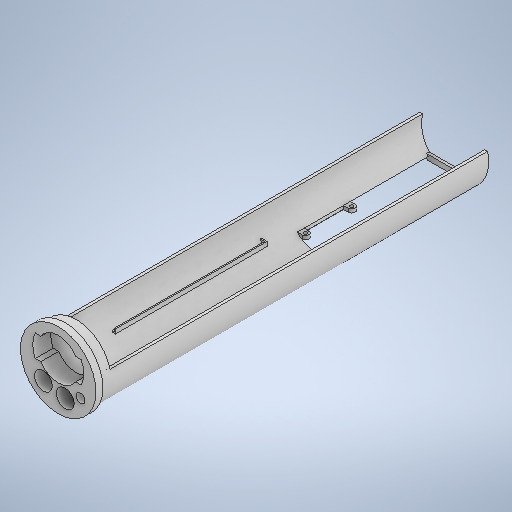
# Autodesk Inventor part: PCB tray CAD
Saved by Autodesk Inventor 2025 (Build 290162000, 162)
## iProperties
Created: 2024-07-01
Part Number: PCB tray CAD
Material: Generic
Document SubType Name: Modeling
Designer: track
Density: 1 g/cm^3
Appearance: Default
Author: track
## iProperties of the stored document PCB tray CAD_3DPrint.ipt
Created: 2024-07-01
Part Number: PCB tray CAD_3DPrint
Material: Generic
Document SubType Name: Modeling
Designer: track
Density: 1 g/cm^3
Appearance: Default
Author: track
Autodesk Inventor part; units mm, degrees
ref_plane "YZ Plane" through (0, 0, 0) normal (1, 0, 0) x (0, 1, 0)
ref_plane "XY Plane" through (0, 0, 0) normal (0, 0, 1) x (1, 0, 0)
sketch "Sketch9" plane through (0, 0, 0) normal (0, 0, 1) x (1, 0, 0)
  circle A0 centre (0, 0) radius 25.4
  circle A1 centre (0, 0) radius 23.4
  dimension "d29" = 50.8
  dimension "d30" = 2
  constraints: 2 centre point, 2 coincident
  measures "d29" diameter of A0
  measures "d30" radial gap between concentric circles of A0 A1
extrude "Extrusion7" add sketch "Sketch9" against normal blind 287
sketch "Sketch10" plane through (0, 0, 0) normal (0, 0, 1) x (1, 0, 0)
  circle A0 centre (-10.795, -12.065) radius 6.5
  circle A1 centre (5.08, -15.24) radius 6.55
  circle A2 centre (16.129, -9.525) radius 3.3
  circle A3 centre (0, 0) radius 23.4 projected
  line L0 (17.25, -1.015) -> (-17.25, -1.015) construction
  line L1 (-17.25, -1.015) -> (-17.25, 14.985) construction
  line L2 (-17.25, 14.985) -> (17.25, 14.985) construction
  line L3 (17.25, 14.985) -> (17.25, -1.015) construction
  line L4 (17.25, -1.015) -> (-17.25, 14.985) construction
  line L5 (-17.25, -1.015) -> (17.25, 14.985) construction
  arc A4 (-12.6886, -1.015) -> (12.6886, -1.015) centre (0, 6.985) ccw
  arc A5 (12.6886, 14.985) -> (-12.6886, 14.985) centre (0, 6.985) ccw
  circle A6 centre (0, 6.985) radius 18.5 construction
  arc A7 (16.6808, -1.015) -> (16.6808, 14.985) centre (0, 6.985) ccw
  arc A8 (-16.6808, 14.985) -> (-16.6808, -1.015) centre (0, 6.985) ccw
  line L6 (-16.6808, 14.985) -> (-12.6886, 14.985)
  line L7 (12.6886, 14.985) -> (16.6808, 14.985)
  line L8 (16.6808, -1.015) -> (12.6886, -1.015)
  line L9 (-12.6886, -1.015) -> (-16.6808, -1.015)
  point P0 (18.5865, 14.2162)
  point P1 (17.7647, -15.2307)
  dimension "d33" = 13
  dimension "d34" = 13.1
  dimension "d35" = 6.6
  dimension "d90" = 16
  dimension "d91" = 34.5
  dimension "d92" = 15
  dimension "d93" = 15
  dimension "d94" = 37
  dimension "d95" = 0
  dimension "d96" = 6.985
  dimension "d97" = 9.525
  dimension "d98" = 16.129
  dimension "d99" = 5.08
  dimension "d100" = 15.24
  dimension "d101" = 10.795
  dimension "d102" = 12.065
  constraints: 20 end point, 12 point on circle, 8 centre point, 8 point on line, 3 collinear, 3 parallel, 2 concentric, 2 midpoint, 1 coincident, 1 horizontal, 1 perpendicular
  measures "d33" diameter of A0
  measures "d34" diameter of A1
  measures "d35" diameter of A2
  measures "d90" distance between parallel lines of L2 L0
  measures "d91" distance of L1.end L2.end
  measures "d92" radius of A5
  measures "d93" radius of A4
  measures "d94" diameter of A6
  measures "d95" horizontal distance of point (0, 0) A4.centre
  measures "d96" distance of A4.centre point (0, 0)
  measures "d97" vertical distance of A2.centre point (0, 0)
  measures "d98" horizontal distance of point (0, 0) A2.centre
  measures "d99" horizontal distance of point (0, 0) A1.centre
  measures "d100" vertical distance of A3.centre A1.centre
  measures "d101" horizontal distance of point (0, 0) A0.centre
  measures "d102" vertical distance of point (0, 0) A0.centre
extrude "Extrusion8" add sketch "Sketch10" against normal blind 13
ref_plane "Work Plane1" through (0, 25.4, 0) normal (0, 1, 0) x (-1, 0, 0)
sketch "Sketch11" plane through (0, 25.4, 0) normal (0, 1, 0) x (-1, 0, 0)
  line L0 (-25.4, -287) -> (25.4, -287) projected
  line L1 (-25.4, 0) -> (-25.4, -287) projected
  line L2 (25.4, -287) -> (-25.4, -287)
  line L3 (-25.4, -287) -> (-25.4, -190)
  line L4 (-25.4, -190) -> (25.4, -190)
  line L5 (25.4, -190) -> (25.4, -287)
  point P0 (0, 0)
  dimension "d53" = 97
  constraints: 8 end point, 2 parallel, 1 horizontal, 1 perpendicular, 1 point on line
  measures "d53" distance of L4.end L0.end
extrude "Extrusion9" cut sketch "Sketch11" against normal blind 19.05
sketch "Sketch12" plane through (0, 0, -287) normal (0, 0, -1) x (-1, 0, 0)
  circle A0 centre (0, 0) radius 25.4 projected
  line L0 (-19.2809, -16.535) -> (19.2809, -16.535)
  line L1 (16, -16.535) -> (-16, -16.535) projected
  arc A1 (-19.2809, -16.535) -> (19.2809, -16.535) centre (0, 0) ccw
  dimension "d86" = 16.535
  constraints: 4 point on circle, 2 end point, 1 centre point, 1 concentric, 1 horizontal
  measures "d86" distance from line of A0.centre L0
extrude "Extrusion10" cut sketch "Sketch12" against normal blind 97 contours L0 A0 picked at (1.0399, -19.4259)
ref_plane "Work Plane3" through (0, -16.51, 0) normal (0, 1, 0) x (-1, 0, 0)
sketch "Sketch13" plane through (0, -16.51, 0) normal (0, 1, 0) x (-1, 0, 0)
  line L0 (0, 0) -> (0, -257.1233) construction
  line L1 (-16.5576, -287) -> (-16.5576, -190) projected
  line L2 (-16.5576, -190) -> (-13.0576, -190)
  line L3 (-13.0576, -190) -> (-13.0576, -195) construction
  line L4 (-13.0576, -195) -> (-16.5576, -195)
  line L5 (-16.5576, -195) -> (-16.5576, -190)
  line L6 (16.5576, -190) -> (16.5576, -287) projected
  line L7 (16.5576, -190) -> (13.0576, -190)
  line L8 (13.0576, -190) -> (13.0576, -195) construction
  line L9 (13.0576, -195) -> (16.5576, -195)
  line L10 (16.5576, -195) -> (16.5576, -190)
  line L11 (-16.5576, -223.5) -> (-13.0576, -223.5)
  line L12 (-13.0576, -223.5) -> (-13.0576, -228.5) construction
  line L13 (-13.0576, -228.5) -> (-16.5576, -228.5)
  line L14 (-16.5576, -228.5) -> (-16.5576, -223.5)
  line L15 (16.5576, -223.5) -> (13.0576, -223.5)
  line L16 (13.0576, -223.5) -> (13.0576, -228.5) construction
  line L17 (13.0576, -228.5) -> (16.5576, -228.5)
  line L18 (16.5576, -228.5) -> (16.5576, -223.5)
  arc A0 (-13.0576, -195) -> (-13.0576, -190) centre (-13.0576, -192.5) ccw
  arc A1 (13.0576, -190) -> (13.0576, -195) centre (13.0576, -192.5) ccw
  arc A2 (-13.0576, -228.5) -> (-13.0576, -223.5) centre (-13.0576, -226) ccw
  arc A3 (13.0576, -223.5) -> (13.0576, -228.5) centre (13.0576, -226) ccw
  circle A4 centre (-13.0576, -192.5) radius 1.25
  circle A5 centre (13.0576, -192.5) radius 1.25
  circle A6 centre (-13.0576, -226) radius 1.25
  circle A7 centre (13.0576, -226) radius 1.25
  point P0 (-10.5576, -192.5)
  point P1 (16.5576, -228.5)
  point P2 (16.5576, -223.5)
  point P3 (-16.5576, -223.5)
  point P4 (-16.5576, -228.5)
  dimension "d60" = 5
  dimension "d61" = 5
  dimension "d62" = 28.5
  dimension "d63" = 6
  dimension "d64" = 2.5
  dimension "d65" = 2.5
  constraints: 34 end point, 9 point on circle, 8 centre point, 8 parallel, 8 tangent, 5 point on line, 4 coincident, 4 horizontal, 4 perpendicular, 1 vertical, 6 other
  measures "d60" distance of L2.end L3.end
  measures "d61" distance of L11.end L12.end
  measures "d62" distance between parallel lines of L4 L11
  measures "d63" distance from line of L1 point (-10.558, -192.5)
  measures "d64" diameter of A4
  measures "d65" diameter of A6
extrude "Extrusion11" add sketch "Sketch13" against normal blind 2.54
sketch "Sketch14" plane through (0, 0, -190) normal (0, 0, -1) x (-1, 0, 0)
  line L0 (16.5576, -19.05) -> (13.5889, -19.05) projected
  arc A0 (-13.5889, -19.05) -> (13.5889, -19.05) centre (0, 0) ccw projected
  line L1 (-13.5889, -19.05) -> (-16.5576, -19.05) projected
  line L2 (-16.5576, -19.05) -> (-16.5576, -16.535) projected
  line L3 (-19.2809, -16.535) -> (-16.5576, -16.535) projected
  arc A1 (-19.2809, -16.535) -> (19.2809, -16.535) centre (0, 0) ccw projected
  line L4 (16.5576, -16.535) -> (19.2809, -16.535) projected
  line L5 (16.5576, -16.535) -> (16.5576, -19.05) projected
  line L6 (13.0576, -16.51) -> (13.0576, -19.05) projected
  line L7 (13.0576, -19.05) -> (16.8005, -19.05)
  line L8 (-13.0576, -16.51) -> (-13.0576, -19.05) projected
  line L9 (-13.0576, -19.05) -> (-16.8005, -19.05)
  point P0 (-16.5576, -19.2615)
  point P1 (16.5576, -19.2615)
  constraints: 4 end point, 4 point on circle, 3 point on line, 1 perpendicular
extrude "Extrusion12" add sketch "Sketch14" along normal up to surface (38.5 mm away) contours L5 L4 A1 L7 | A1 L3 L2 L9
sketch "Sketch15" plane through (0, 25.4, 0) normal (0, 1, 0) x (-1, 0, 0)
  line L0 (-25.4, 0) -> (-25.4, -287) projected
  line L1 (25.4, 0) -> (25.4, -287) projected
  line L2 (-25.4, -13) -> (25.4, -13)
  line L3 (25.4, -13) -> (25.4, -193)
  line L4 (25.4, -193) -> (-25.4, -193)
  line L5 (-25.4, -193) -> (-25.4, -13)
  line L6 (23.4, -13) -> (-23.4, -13) projected
  point P0 (0, 0)
  point P1 (-25.4, -193)
  point P2 (25.4, -13)
  dimension "d70" = 0
  dimension "d71" = 180
  constraints: 8 end point, 2 parallel, 2 point on line, 1 horizontal, 1 perpendicular
  measures "d70" distance between parallel lines of L6 L2
  measures "d71" distance between parallel lines of L2 L4
extrude "Extrusion13" cut sketch "Sketch15" against normal up to surface (19.05 mm away)
sketch "Sketch17" plane through (0, 0, -287) normal (0, 0, -1) x (-1, 0, 0)
  circle A0 centre (0, 0) radius 25.4
  arc A1 (-16.8005, -19.05) -> (16.8005, -19.05) centre (0, 0) ccw projected
  line L0 (-19.2809, -16.535) -> (-16.5576, -16.535) projected
  line L1 (-20.32, -15.24) -> (20.32, -15.24)
  line L2 (16.5576, -19.05) -> (13.0576, -19.05) projected
  line L3 (-16.8005, -19.05) -> (16.8005, -19.05)
  point P0 (16.8005, -19.05)
  dimension "d74" = 3.81
  constraints: 4 end point, 2 parallel, 2 point on circle, 1 centre point, 1 coincident, 1 concentric
  measures "d74" distance between parallel lines of L1 L3
extrude "Extrusion14" add sketch "Sketch17" against normal blind 2 contours L1 A0 L3 L2
sketch "Sketch18" plane through (0, 0, -13) normal (0, 0, -1) x (-1, 0, 0)
  circle A0 centre (0, 0) radius 27.4
  circle A1 centre (0, 0) radius 25.4
  arc A2 (16.8005, -19.05) -> (24.5934, 6.35) centre (0, 0) ccw projected
  dimension "d87" = 2
  constraints: 2 centre point, 2 coincident, 1 concentric
  measures "d87" radial gap between concentric circles of A0 A1
extrude "Extrusion15" add sketch "Sketch18" along normal blind 5 from surface at -13
sketch "Sketch20" plane through (0, 0, -13) normal (0, 0, -1) x (-1, 0, 0)
  arc A0 (-22.5219, 6.35) -> (-17.7568, -15.24) centre (0, 0) ccw projected
  line L0 (-20.4714, -11.335) -> (20.4714, -11.335) construction
  arc A1 (-22.5219, 6.35) -> (22.5219, 6.35) centre (0, 0) ccw projected
  arc A2 (24.5934, 6.35) -> (-24.5934, 6.35) centre (0, 0) ccw projected
  line L1 (0, -23.4) -> (0, 25.4) construction
  line L2 (-16.4531, -11.335) -> (-17.3421, -11.335)
  line L3 (-17.3421, -11.335) -> (-17.3421, -13.621)
  line L4 (-17.3421, -13.621) -> (-19.027, -13.621)
  line L5 (-16.4531, -11.335) -> (-16.4531, -14.51)
  line L6 (-16.4531, -14.51) -> (-18.3581, -14.51)
  circle A3 centre (0, 0) radius 23.4
  line L7 (20.4714, -11.335) -> (-20.4714, -11.335) construction
  line L8 (16.4531, -11.335) -> (17.3421, -11.335)
  line L9 (17.3421, -11.335) -> (17.3421, -13.621)
  line L10 (17.3421, -13.621) -> (19.027, -13.621)
  line L11 (16.4531, -11.335) -> (16.4531, -14.51)
  line L12 (16.4531, -14.51) -> (18.3581, -14.51)
  arc A4 (-13.5889, -19.05) -> (13.5889, -19.05) centre (0, 0) ccw projected
  point P0 (19.027, -13.621)
  point P1 (-19.027, -13.621)
  dimension "d111" = 1.905
  dimension "d112" = 0.889
  dimension "d113" = 3.175
  dimension "d114" = 0.889
  dimension "d126" = 8.89
  dimension "d127" = 34.6842
  constraints: 26 end point, 8 symmetric about line, 4 point on line, 3 point on circle, 3 vertical, 2 perpendicular, 1 centre point, 1 coincident, 1 concentric, 1 horizontal, 5 other
  measures "d111" distance of L5.end L6.end
  measures "d112" distance of L2.start L2.end
  measures "d113" distance of L2.start L5.end
  measures "d114" distance between parallel lines of L6 L4
  measures "d126" distance from line of point (0, -23.4) L6
  measures "d127" distance between parallel lines of L9 L3
extrude "Extrusion16" add sketch "Sketch20" along normal blind 155 contours L4 L3 L2 L5 L6 A0 | A1 L12 L11 L8 L9 L10
sketch "Sketch21" plane through (0, 0, -13) normal (0, 0, -1) x (-1, 0, 0)
  circle A0 centre (0, 0) radius 23.4
  arc A1 (24.5934, 6.35) -> (-24.5934, 6.35) centre (0, 0) ccw projected
  arc A2 (-13.5889, -19.05) -> (13.5889, -19.05) centre (0, 0) ccw projected
  constraints: 1 centre point, 1 coincident, 1 concentric
extrude "Extrusion17" cut sketch "Sketch21" along normal blind 45
sketch "Sketch23" plane through (0, 0, -58) normal (0, 0, 1) x (1, 0, 0)
  circle A0 centre (0, 0) radius 23.4
  arc A1 (-22.5219, 6.35) -> (-17.7568, -15.24) centre (0, 0) ccw projected
  line L0 (-17.3421, -13.621) -> (-17.3421, -11.335) projected
  line L1 (-17.3421, -11.335) -> (-17.3421, -13.621)
  line L2 (-17.3421, -13.621) -> (-19.027, -13.621)
  line L3 (-17.3421, -11.335) -> (-20.4714, -11.335)
  arc A2 (-13.5889, -19.05) -> (13.5889, -19.05) centre (0, 0) ccw projected
  line L4 (0, -23.4) -> (0, 23.4) construction
  line L5 (17.3421, -13.621) -> (17.3421, -11.335)
  line L6 (17.3421, -13.621) -> (19.027, -13.621)
  line L7 (17.3421, -11.335) -> (20.4714, -11.335)
  point P0 (-19.027, -13.621)
  point P1 (19.027, -13.621)
  dimension "d120" = 0
  constraints: 14 end point, 4 point on circle, 4 symmetric about line, 2 vertical, 1 centre point, 1 coincident, 1 concentric, 1 horizontal, 1 perpendicular
  measures "d120" distance from line of point (0, 0) L4
extrude "Extrusion18" add sketch "Sketch23" along normal blind 1 from surface at -110 contours A0 L6 L5 L7 | L3 L0 L2 A0
sketch "Sketch27" plane through (0, 0, -13) normal (0, 0, -1) x (-1, 0, 0)
  line L0 (-22.5219, 6.35) -> (-24.5934, 6.35) projected
  line L1 (-23.5577, 6.35) -> (-23.5577, 9.4971) construction
  circle A0 centre (0, 0) radius 25.4 projected
  circle A1 centre (-23.5577, 6.85) radius 0.5
  line L2 (0, 25.4) -> (0, -23.4) construction
  arc A2 (-13.5889, -19.05) -> (13.5889, -19.05) centre (0, 0) ccw projected
  circle A3 centre (23.5577, 6.85) radius 0.5
  dimension "d136" = 1
  dimension "d137" = 0.5
  dimension "d138" = 0
  constraints: 4 end point, 3 point on circle, 2 centre point, 2 vertical, 1 midpoint, 1 point on line, 1 symmetric about line, 1 other
  measures "d136" diameter of A1
  measures "d137" distance from line of L0 A1.centre
  measures "d138" distance from line of point (0, 0) L2
extrude "Extrusion20" cut sketch "Sketch27" against normal blind 2 contours A1 | A3
sketch "Sketch28" plane through (17.3421, -13.621, -58) normal (0, 1, 0) x (1, 0, 0)
  line L0 (0, 0) -> (0, 109) projected
  line L1 (1.6849, 109) -> (1.6849, 0) projected
  line L2 (0, 109) -> (1.6849, 109)
  line L3 (1.6849, 109) -> (1.6849, 107.3236)
  line L4 (1.6849, 107.3236) -> (0, 107.3236)
  line L5 (0, 107.3236) -> (0, 109)
  line L6 (-18.8121, -45) -> (-5.7121, -45) projected
  line L7 (-18.8121, -45) -> (-18.8121, -58) construction
  line L8 (-18.8121, -45) -> (-18.8121, -58) projected
  point P0 (-17.3421, -58)
  point P1 (0, 107.3236)
  dimension "d141" = 1.6849
  dimension "d142" = 1.6764
  constraints: 10 end point, 2 parallel, 2 point on line, 1 horizontal, 1 perpendicular
  measures "d141" distance of L0.end L2.end
  measures "d142" distance between parallel lines of L2 L4
extrude "Extrusion21" cut sketch "Sketch28" against normal blind 1
sketch "Sketch29" plane through (-19.027, -13.621, -58) normal (0, 1, 0) x (1, 0, 0)
  line L0 (1.6849, 109) -> (-1.4443, 109) projected
  line L1 (0, 0) -> (0, 109) projected
  line L2 (1.6849, 109) -> (0, 109)
  line L3 (0, 109) -> (0, 107.3236)
  line L4 (0, 107.3236) -> (1.6849, 107.3236)
  line L5 (1.6849, 107.3236) -> (1.6849, 109)
  point P0 (19.027, -58)
  dimension "d145" = 1.6764
  constraints: 8 end point, 2 parallel, 1 horizontal, 1 perpendicular, 1 point on line
  measures "d145" distance between parallel lines of L0 L4
extrude "Extrusion22" cut sketch "Sketch29" against normal blind 1
body "Solid2"
